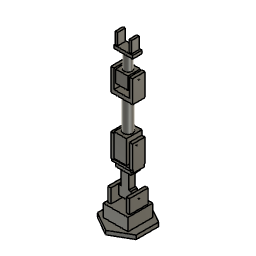
robot_arm (Autodesk Fusion 360 design; units mm, degrees)
Autodesk Fusion 360 part; units mm, degrees
sketch "Sketch1" plane through (0, 0, 0) normal (0, 0, 1) x (1, 0, 0)
  line L0 (125, 72.1688) -> (0, 144.3376)
  line L1 (0, 144.3376) -> (-125, 72.1688)
  line L2 (-125, 72.1688) -> (-125, -72.1688)
  line L3 (-125, -72.1688) -> (0, -144.3376)
  line L4 (0, -144.3376) -> (125, -72.1688)
  line L5 (125, -72.1688) -> (125, 72.1688)
extrude "Extrude1" add sketch "Sketch1" along normal blind 25 makes body 1
sketch "Sketch2" plane through (0, 0, 25) normal (0, 0, 1) x (-1, 0, 0)
  line L0 (-125, 72.1688) -> (-125, -72.1688)
  line L1 (-125, -72.1688) -> (0, -144.3376)
  line L2 (0, -144.3376) -> (125, -72.1688)
  line L3 (125, -72.1688) -> (125, 72.1688)
  line L4 (125, 72.1688) -> (0, 144.3376)
  line L5 (0, 144.3376) -> (-125, 72.1688)
  line L6 (80, -80) -> (-80, -80)
  line L7 (-80, -80) -> (-80, 80)
  line L8 (-80, 80) -> (80, 80)
  line L9 (80, 80) -> (80, -80)
  constraint horizontal L6
  constraint vertical L7
  constraint horizontal L8
  constraint vertical L9
extrude "Extrude2" add sketch "Sketch2" along normal blind 80 contours L6 L7 L8 L9 bodies 1
sketch "Sketch3" plane through (0, 0, 105) normal (0, 0, 1) x (-1, 0, 0)
  line L0 (80, 80) -> (-80, 80)
  line L1 (-80, 80) -> (-80, -80)
  line L2 (-80, -80) -> (80, -80)
  line L3 (80, -80) -> (80, 80)
  line L4 (-70, 60) -> (-50, 60)
  line L5 (-50, 60) -> (-50, -60)
  line L6 (-50, -60) -> (-70, -60)
  line L7 (-70, -60) -> (-70, 60)
  line L8 (40, 60) -> (60, 60)
  line L9 (60, 60) -> (60, -60)
  line L10 (60, -60) -> (40, -60)
  line L11 (40, -60) -> (40, 60)
  constraint horizontal L4
  constraint vertical L5
  constraint horizontal L6
  constraint vertical L7
  constraint horizontal L8
  constraint vertical L9
  constraint horizontal L10
  constraint vertical L11
extrude "Extrude3" add sketch "Sketch3" along normal blind 90 contours L4 L5 L6 L7 | L8 L9 L10 L11 bodies 1
sketch "Sketch5" plane through (-60, 0, 0) normal (-1, 0, 0) x (0, -1, 0)
  line L0 (-60, 105) -> (60, 105)
  line L1 (60, 105) -> (60, 195)
  line L2 (60, 195) -> (-60, 195)
  line L3 (-60, 195) -> (-60, 105)
  circle A0 centre (0, 165) radius 4
  dimension "d9" = 8
  measures "d9" diameter of A0
extrude "Extrude5" cut sketch "Sketch5" against normal blind 140 contours A0 bodies 1
sketch "Sketch6" plane through (0, 0, 0) normal (1, 0, 0) x (0, 1, 0)
  line L0 (20, 180) -> (-20, 180)
  line L1 (-20, 180) -> (-20, 140)
  line L2 (-20, 140) -> (20, 140)
  line L3 (20, 140) -> (20, 180)
  constraint horizontal L0
  constraint vertical L1
  constraint horizontal L2
  constraint vertical L3
move_face "MoveFace1" by (-10, 0, 0) 5 faces at (-46.6667, -60, 135) (-60, 0.0996, 123.6704) (-46.6667, -20, 195) (-40, -0.0996, 123.6704) (-53.3333, 60, 135) on bodies 1
sketch "Sketch8" plane through (0, 80, 0) normal (0, 1, 0) x (-1, 0, 0)
  line L0 (-80, 25) -> (80, 25)
  line L1 (80, 25) -> (80, 105)
  line L2 (80, 105) -> (-80, 105)
  line L3 (-80, 105) -> (-80, 25)
  line L4 (-40, 140) -> (40, 140)
  line L5 (40, 140) -> (40, 200)
  line L6 (40, 200) -> (-40, 200)
  line L7 (-40, 200) -> (-40, 140)
  constraint horizontal L4
  constraint vertical L5
  constraint horizontal L6
  constraint vertical L7
extrude "Extrude7" add sketch "Sketch8" along normal blind 40 separate body contours L4 L5 L6 L7 makes body 2
move_body "Move2" bodies 2 to x (1, 0, 0) y (0, 1, 0) z (0, 0, 1) at (0, -100, 0)
sketch "Sketch9" plane through (0, 0, 200) normal (0, 0, 1) x (-1, 0, 0)
  line L0 (40, 20) -> (-40, 20)
  line L1 (-40, 20) -> (-40, -20)
  line L2 (-40, -20) -> (40, -20)
  line L3 (40, -20) -> (40, 20)
  line L4 (-25.0104, 20) -> (25.3837, 20)
  line L5 (25.3837, 20) -> (25.3837, -20)
  line L6 (25.3837, -20) -> (-25.0104, -20)
  line L7 (-25.0104, -20) -> (-25.0104, 20)
  constraint horizontal L4
  constraint vertical L5
  constraint horizontal L6
  constraint vertical L7
  constraint coincident L2 L5.end
  constraint coincident L0 L4.start
extrude "Extrude8" add sketch "Sketch9" along normal blind 100 contours L0 L2 L4 L5 L6 L7 bodies 2
sketch "Sketch10" plane through (0, 0, 300) normal (0, 0, 1) x (-1, 0, 0)
  line L0 (-25.0104, -20) -> (25.3837, -20)
  line L1 (25.3837, -20) -> (25.3837, 20)
  line L2 (25.3837, 20) -> (-25.0104, 20)
  line L3 (-25.0104, 20) -> (-25.0104, -20)
  line L4 (50, -30) -> (-50, -30)
  line L5 (-50, -30) -> (-50, 30)
  line L6 (-50, 30) -> (50, 30)
  line L7 (50, 30) -> (50, -30)
  line L8 (50, -30) -> (-50, 30) construction
  line L9 (-50, -30) -> (50, 30) construction
  constraint horizontal L4
  constraint perpendicular L4 L5
  constraint parallel L4 L6
  constraint parallel L5 L7
  constraint coincident L8 origin
  constraint coincident L9 origin
extrude "Extrude9" add sketch "Sketch10" along normal blind 25 contours L0 L1 L2 L3 | L4 L5 L6 L7 bodies 2
sketch "Sketch11" plane through (0, 0, 325) normal (0, 0, 1) x (-1, 0, 0)
  line L0 (50, 30) -> (-50, 30)
  line L1 (-50, 30) -> (-50, -30)
  line L2 (-50, -30) -> (50, -30)
  line L3 (50, -30) -> (50, 30)
  line L4 (70, 35) -> (-70, 35)
  line L5 (-70, 35) -> (-70, -35)
  line L6 (-70, -35) -> (70, -35)
  line L7 (70, -35) -> (70, 35)
  line L8 (70, 35) -> (-70, -35) construction
  line L9 (-70, 35) -> (70, -35) construction
  constraint horizontal L4
  constraint perpendicular L4 L5
  constraint parallel L4 L6
  constraint parallel L5 L7
  constraint coincident L8 origin
  constraint coincident L9 origin
extrude "Extrude10" add sketch "Sketch11" along normal blind 15 contours L0 L1 L2 L3 | L4 L5 L6 L7 bodies 2
sketch "Sketch12" plane through (0, 0, 340) normal (0, 0, 1) x (-1, 0, 0)
  line L0 (70, -35) -> (70, 35)
  line L1 (70, 35) -> (-70, 35)
  line L2 (-70, 35) -> (-70, -35)
  line L3 (-70, -35) -> (70, -35)
  line L4 (50, 40) -> (70, 40)
  line L5 (70, 40) -> (70, -40)
  line L6 (70, -40) -> (50, -40)
  line L7 (50, -40) -> (50, 40)
  line L8 (-70, 40) -> (-50, 40)
  line L9 (-50, 40) -> (-50, -40)
  line L10 (-50, -40) -> (-70, -40)
  line L11 (-70, -40) -> (-70, 40)
  constraint horizontal L4
  constraint vertical L5
  constraint horizontal L6
  constraint vertical L7
  constraint horizontal L8
  constraint vertical L9
  constraint horizontal L10
  constraint vertical L11
extrude "Extrude11" add sketch "Sketch12" along normal blind 150 contours L0 L1 L3 L5 L7 | L3 L5 L6 L7 | L1 L4 L5 L7 | L3 L9 L10 L11 | L1 L2 L3 L9 L11 | L1 L8 L9 L11 bodies 2
sketch "Sketch13" plane through (0, 0, 0) normal (0, 1, 0) x (1, 0, 0)
  line L0 (-40, -510) -> (40, -510)
  line L1 (40, -510) -> (40, -360)
  line L2 (40, -360) -> (-40, -360)
  line L3 (-40, -360) -> (-40, -510)
  constraint horizontal L0
  constraint vertical L1
  constraint horizontal L2
  constraint vertical L3
extrude "Extrude12" add sketch "Sketch13" along normal blind 50 and the other way blind 50 separate body makes body 3
sketch "Sketch14" plane through (0, 0, 510) normal (0, 0, 1) x (-1, 0, 0)
  line L0 (-40, 50) -> (-40, -50)
  line L1 (-40, -50) -> (40, -50)
  line L2 (40, -50) -> (40, 50)
  line L3 (40, 50) -> (-40, 50)
  circle A0 centre (0, 0) radius 30
  dimension "d28" = 60
  constraint coincident A0.centre origin
  measures "d28" diameter of A0
extrude "Extrude13" add sketch "Sketch14" along normal blind 200 separate body contours A0 makes body 4
sketch "Sketch15" plane through (0, 0, 710) normal (0, 0, 1) x (-1, 0, 0)
  circle A0 centre (0, 0) radius 30
  line L0 (-70, 40) -> (70, 40)
  line L1 (70, 40) -> (70, -40)
  line L2 (70, -40) -> (-70, -40)
  line L3 (-70, -40) -> (-70, 40)
  line L4 (-70, 40) -> (70, -40) construction
  line L5 (70, 40) -> (-70, -40) construction
  constraint horizontal L0
  constraint perpendicular L0 L1
  constraint parallel L0 L2
  constraint parallel L1 L3
  constraint coincident L4 A0.centre
  constraint coincident L5 A0.centre
  constraint coincident A0.centre origin
extrude "Extrude14" add sketch "Sketch15" along normal blind 25 contours A0 | L0 L1 L2 L3 bodies 4
sketch "Sketch16" plane through (0, 0, 735) normal (0, 0, 1) x (-1, 0, 0)
  line L0 (-70, -40) -> (70, -40)
  line L1 (70, -40) -> (70, 40)
  line L2 (70, 40) -> (-70, 40)
  line L3 (-70, 40) -> (-70, -40)
  line L4 (-50, 40) -> (-50, -40)
  line L5 (50, 40) -> (50, -40)
  constraint coincident L2 L4.start
  constraint coincident L0 L4.end
  constraint perpendicular L0 L4
  constraint coincident L2 L5.start
  constraint coincident L0 L5.end
  constraint perpendicular L2 L5
extrude "Extrude15" add sketch "Sketch16" along normal blind 120 contours L0 L2 L3 L4 | L0 L1 L2 L5 bodies 4
sketch "Sketch17" plane through (0, 0, 855) normal (0, 0, 1) x (-1, 0, 0)
  line L0 (-70, 40) -> (-70, -40)
  line L1 (-70, -40) -> (-50, -40)
  line L2 (-50, -40) -> (-50, 40)
  line L3 (-50, 40) -> (-70, 40)
  line L4 (40, -40) -> (-40, -40)
  line L5 (-40, -40) -> (-40, 40)
  line L6 (-40, 40) -> (40, 40)
  line L7 (40, 40) -> (40, -40)
  constraint horizontal L4
  constraint vertical L5
  constraint horizontal L6
  constraint vertical L7
extrude "Extrude16" add sketch "Sketch17" against normal blind 80 separate body contours L4 L5 L6 L7 makes body 5
sketch "Sketch18" plane through (0, 0, 855) normal (0, 0, 1) x (-1, 0, 0)
  line L0 (40, 40) -> (-40, 40)
  line L1 (-40, 40) -> (-40, -40)
  line L2 (-40, -40) -> (40, -40)
  line L3 (40, -40) -> (40, 40)
  circle A0 centre (0, 0) radius 25.6139
  constraint coincident A0.centre origin
extrude "Extrude17" add sketch "Sketch18" along normal blind 100 contours A0 bodies 5
sketch "Sketch19" plane through (0, 0, 955) normal (0, 0, 1) x (-1, 0, 0)
  circle A0 centre (0, 0) radius 25.6139
  line L0 (-60, 30) -> (60, 30)
  line L1 (60, 30) -> (60, -30)
  line L2 (60, -30) -> (-60, -30)
  line L3 (-60, -30) -> (-60, 30)
  constraint horizontal L0
  constraint vertical L1
  constraint horizontal L2
  constraint vertical L3
extrude "Extrude18" add sketch "Sketch19" along normal blind 20 separate body contours A0 | L0 L1 L2 L3 makes body 6
sketch "Sketch20" plane through (0, 0, 975) normal (0, 0, 1) x (-1, 0, 0)
  line L0 (-60, -30) -> (60, -30)
  line L1 (60, -30) -> (60, 30)
  line L2 (60, 30) -> (-60, 30)
  line L3 (-60, 30) -> (-60, -30)
  line L4 (55, 25) -> (40, 25)
  line L5 (40, 25) -> (40, -25)
  line L6 (40, -25) -> (55, -25)
  line L7 (55, -25) -> (55, 25)
  line L8 (-55, 25) -> (-40, 25)
  line L9 (-40, 25) -> (-40, -25)
  line L10 (-40, -25) -> (-55, -25)
  line L11 (-55, -25) -> (-55, 25)
  constraint horizontal L4
  constraint vertical L5
  constraint horizontal L6
  constraint vertical L7
  constraint horizontal L8
  constraint vertical L9
  constraint horizontal L10
  constraint vertical L11
extrude "Extrude19" add sketch "Sketch20" along normal blind 75 separate body contours L4 L5 L6 L7 | L8 L9 L10 L11 makes body 7 at (40, -8.3333, 1000) makes body 8 at (-55, 8.3333, 1025)
sketch "Sketch21" plane through (-70, 0, 0) normal (-1, 0, 0) x (0, -1, 0)
  circle A0 centre (0, 165) radius 4
  line L0 (-60, 105) -> (60, 105)
  line L1 (60, 105) -> (60, 195)
  line L2 (60, 195) -> (-60, 195)
  line L3 (-60, 195) -> (-60, 105)
  circle A1 centre (0, 165) radius 4
  constraint concentric A0 A1
extrude "Extrude20" cut sketch "Sketch21" against normal blind 160 contours A0 A1 bodies 2
sketch "Sketch22" plane through (-70, 0, 0) normal (-1, 0, 0) x (0, -1, 0)
  line L0 (-35, 325) -> (35, 325)
  line L1 (35, 325) -> (35, 340)
  line L2 (35, 340) -> (40, 340)
  line L3 (40, 340) -> (40, 490)
  line L4 (40, 490) -> (-40, 490)
  line L5 (-40, 490) -> (-40, 340)
  line L6 (-40, 340) -> (-35, 340)
  line L7 (-35, 340) -> (-35, 325)
  circle A0 centre (15, 470) radius 4
  dimension "d45" = 8
  measures "d45" diameter of A0
extrude "Extrude21" cut sketch "Sketch22" against normal blind 160 contours A0 bodies 2 3
sketch "Sketch23" plane through (-70, 0, 0) normal (-1, 0, 0) x (0, -1, 0)
  line L0 (-40, 710) -> (40, 710)
  line L1 (40, 710) -> (40, 855)
  line L2 (40, 855) -> (-40, 855)
  line L3 (-40, 855) -> (-40, 710)
  circle A0 centre (0, 830) radius 4
  dimension "d48" = 8
  measures "d48" diameter of A0
extrude "Extrude22" cut sketch "Sketch23" against normal blind 240 contours A0 bodies 4 8 7 5 6
copy_body "Body->Comp22" bodies 6 removing the originals makes body 9 in component "old_component (1)"
copy_body "Body->Comp23" bodies 7 removing the originals makes body 10 in component "old_component (2)"
copy_body "Body->Comp24" bodies 8 removing the originals makes body 11 in component "old_component (3)"
copy_body "Body->Comp25" bodies 5 removing the originals makes body 12 in component "old_component (4)"
copy_body "Body->Comp26" bodies 4 removing the originals makes body 13 in component "old_component (5)"
copy_body "Body->Comp27" bodies 3 removing the originals makes body 14 in component "old_component (6)"
copy_body "Body->Comp28" bodies 2 removing the originals makes body 15 in component "old_component (7)"
copy_body "Body->Comp29" bodies 1 removing the originals makes body 16 in component "old_component"
copy_body "CopyPasteBodies1" bodies 9 makes body 17 in component "hand_link_1"
copy_body "CopyPasteBodies1'" bodies 10 body 10 seen with x (1, 0, 0) y (0, 1, 0) z (0, 0, 1) at (-7.5, 0, 0) makes body 18 in component "tump_link_1"
copy_body "CopyPasteBodies1''" bodies 11 body 11 seen with x (1, 0, 0) y (0, 1, 0) z (0, 0, 1) at (-2.5, 0, 0) makes body 19 in component "finger_link_1"
copy_body "CopyPasteBodies1'''" bodies 12 makes body 20 in component "wrist_link_1"
copy_body "CopyPasteBodies1''''" bodies 13 makes body 21 in component "under_arm_link_1"
copy_body "CopyPasteBodies1'''''" bodies 14 makes body 22 in component "elbow_link_1"
copy_body "CopyPasteBodies1''''''" bodies 15 makes body 23 in component "upper_arm_link_1"
copy_body "CopyPasteBodies1'''''''" bodies 16 makes body 24 in component "base_link"
component "old_component (1)" placed x (1, 0, 0) y (0, 1, 0) z (0, 0, 1) at (0, 0, 0)
component "old_component (2)" placed x (1, 0, 0) y (0, 1, 0) z (0, 0, 1) at (-7.5, 0, 0)
component "old_component (3)" placed x (1, 0, 0) y (0, 1, 0) z (0, 0, 1) at (-2.5, 0, 0)
component "old_component (4)" placed x (1, 0, 0) y (0, 1, 0) z (0, 0, 1) at (0, 0, 0)
component "old_component (5)" placed x (1, 0, 0) y (0, 1, 0) z (0, 0, 1) at (0, 0, 0)
component "old_component (6)" placed x (1, 0, 0) y (0, 1, 0) z (0, 0, 1) at (0, 0, 0)
component "old_component (7)" placed x (1, 0, 0) y (0, 1, 0) z (0, 0, 1) at (0, 0, 0)
component "old_component" placed x (1, 0, 0) y (0, 1, 0) z (0, 0, 1) at (0, 0, 0)
component "hand_link_1" placed x (1, 0, 0) y (0, 1, 0) z (0, 0, 1) at (0, 0, 0)
component "tump_link_1" placed x (1, 0, 0) y (0, 1, 0) z (0, 0, 1) at (0, 0, 0)
component "finger_link_1" placed x (1, 0, 0) y (0, 1, 0) z (0, 0, 1) at (0, 0, 0)
component "wrist_link_1" placed x (1, 0, 0) y (0, 1, 0) z (0, 0, 1) at (0, 0, 0)
component "under_arm_link_1" placed x (1, 0, 0) y (0, 1, 0) z (0, 0, 1) at (0, 0, 0)
component "elbow_link_1" placed x (1, 0, 0) y (0, 1, 0) z (0, 0, 1) at (0, 0, 0)
component "upper_arm_link_1" placed x (1, 0, 0) y (0, 1, 0) z (0, 0, 1) at (0, 0, 0)
component "base_link" placed x (1, 0, 0) y (0, 1, 0) z (0, 0, 1) at (0, 0, 0)
named bodies: "base_link", "upper_arm_link", "elbow_link", "under_arm_link", "wrist_link", "tump_link", "finger_link", "hand_link"
